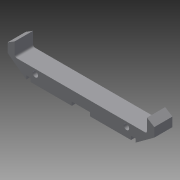
# Autodesk Inventor part: base
Saved by Autodesk Inventor 2014 SP1 (Build 180222100, 222)
## iProperties
Created: 2014-09-21
Part Number: base
Material: Générique
Document SubType Name: Modeling
Designer: astralien3000
Density: 1 g/cm^3
Appearance: Par défaut
Author: astralien3000
Autodesk Inventor part; units mm, degrees
ref_plane "YZ Plane" through (0, 0, 0) normal (1, 0, 0) x (0, 1, 0)
ref_plane "XZ Plane" through (0, 0, 0) normal (0, 1, 0) x (-1, 0, 0)
ref_plane "XY Plane" through (0, 0, 0) normal (0, 0, 1) x (1, 0, 0)
sketch "Esquisse1" plane through (0, 0, 0) normal (0, 1, 0) x (-1, 0, 0)
  circle A0 centre (0, 0) radius 25 construction
  line L0 (-25, 0) -> (25, 0) construction
  arc A1 (-75, -80.7775) -> (-75, 80.7775) centre (-25, 0) ccw construction
  arc A2 (75, 80.7775) -> (75, -80.7775) centre (25, 0) ccw construction
  line L1 (0, 25) -> (0, 0) construction
  line L2 (-75, 80.7775) -> (75, 80.7775)
  line L3 (-75, -80.7775) -> (75, -80.7775)
  arc A3 (75, -80.7775) -> (75, 80.7775) centre (25, 0) ccw
  arc A4 (-75, 80.7775) -> (-75, -80.7775) centre (-25, 0) ccw
  dimension "d0" = 50
  dimension "d1" = 190
  dimension "d2" = 150
  constraints: 11 point on circle, 8 end point, 5 centre point, 3 coincident, 2 perpendicular, 1 horizontal, 1 midpoint, 2 other
  measures "d0" diameter of A0
  measures "d1" diameter of A1
  measures "d2" distance of L2.start L2.end
extrude "Extrusion1" add sketch "Esquisse1" along normal mid plane 20
sketch "Esquisse4" plane through (0, -10, 0) normal (0, -1, 0) x (1, 0, 0)
  line L0 (-50, 40) -> (50, 40) construction
  line L1 (50, 40) -> (50, -40) construction
  line L2 (50, -40) -> (-50, -40) construction
  line L3 (-50, -40) -> (-50, 40) construction
  circle A0 centre (-50, 40) radius 3
  circle A1 centre (50, 40) radius 3
  circle A2 centre (50, -40) radius 3
  circle A3 centre (-50, -40) radius 3
  line L4 (75, 80.7775) -> (-75, 80.7775) projected
  point P0 (0, 0)
  dimension "d15" = 80
  dimension "d16" = 100
  dimension "d17" = 50
  dimension "d18" = 40
  dimension "d19" = 6
  dimension "d20" = 6
  dimension "d21" = 6
  dimension "d22" = 6
  dimension "d25" = 40.7775
  constraints: 8 end point, 4 centre point, 4 coincident, 2 parallel, 1 horizontal, 1 perpendicular
  measures "d15" distance of L0.end L1.end
  measures "d16" distance of L0.start L0.end
  measures "d17" distance from line of L1 point (0, 0)
  measures "d18" distance from line of L2 point (0, 0)
  measures "d19" diameter of A0
  measures "d20" diameter of A1
  measures "d21" diameter of A2
  measures "d22" diameter of A3
  measures "d25" distance between parallel lines of L4 L0
extrude "Extrusion4" cut sketch "Esquisse4" against normal through all
sketch "Esquisse12" plane through (0, -10, 0) normal (0, -1, 0) x (1, 0, 0)
  circle A0 centre (50, -40) radius 3 projected
  circle A1 centre (-50, 40) radius 3 projected
  circle A2 centre (50, 40) radius 3 projected
  circle A3 centre (-50, -40) radius 3 projected
  line L0 (75, 80.7775) -> (-75, 80.7775) projected
  arc A4 (-75, 80.7775) -> (-75, -80.7775) centre (-25, 0) ccw projected
  line L1 (-75, -80.7775) -> (75, -80.7775) projected
  arc A5 (75, -80.7775) -> (75, 80.7775) centre (25, 0) ccw projected
  line L2 (-72.5, 60) -> (72.5, 60)
  line L3 (72.5, 60) -> (72.5, 45)
  line L4 (72.5, 45) -> (-72.5, 45)
  line L5 (-72.5, 45) -> (-72.5, 60)
  line L6 (-60, 45) -> (60, 45)
  line L7 (60, 45) -> (60, 30)
  line L8 (60, 30) -> (-60, 30)
  line L9 (-60, 30) -> (-60, 45)
  line L10 (-72.5, 45) -> (-80.5, 45)
  line L11 (-80.5, 45) -> (-80.5, 55)
  line L12 (-80.5, 55) -> (-72.5, 55)
  line L13 (-72.5, 55) -> (-72.5, 45)
  line L14 (72.5, 45) -> (80.5, 45)
  line L15 (80.5, 45) -> (80.5, 55)
  line L16 (80.5, 55) -> (72.5, 55)
  line L17 (72.5, 55) -> (72.5, 45)
  line L18 (-60, 30) -> (-80.5, 45)
  line L19 (60, 30) -> (80.5, 45)
  line L20 (-80.5, 55) -> (-72.5, 60)
  line L21 (-72.5, 55) -> (-72.5, 60)
  line L22 (80.5, 55) -> (72.5, 60)
  line L23 (72.5, 60) -> (72.5, 55)
  line L24 (-60, 30) -> (-55, 30)
  line L25 (-55, 30) -> (-55, 34)
  line L26 (-55, 34) -> (-60, 34)
  line L27 (-60, 34) -> (-60, 30)
  line L28 (60, 30) -> (55, 30)
  line L29 (55, 30) -> (55, 34)
  line L30 (55, 34) -> (60, 34)
  line L31 (60, 34) -> (60, 30)
  line L32 (10, 30) -> (-10, 30)
  line L33 (-10, 30) -> (-10, 34)
  line L34 (-10, 34) -> (10, 34)
  line L35 (10, 34) -> (10, 30)
  point P0 (0, 0)
  dimension "d101" = 145
  dimension "d102" = 15
  dimension "d103" = 40.7775
  dimension "d105" = 72.5
  dimension "d106" = 10
  dimension "d107" = 10
  dimension "d108" = 10
  dimension "d109" = 8
  dimension "d110" = 8
  dimension "d111" = 5
  dimension "d112" = 5
  dimension "d116" = 5
  dimension "d117" = 4
  dimension "d118" = 5
  dimension "d119" = 4
  dimension "d120" = 4
  dimension "d121" = 20
  dimension "d122" = 10
  dimension "d144" = 5
  constraints: 68 end point, 15 parallel, 7 horizontal, 7 perpendicular, 2 point on line, 1 collinear
  measures "d101" distance of L2.start L2.end
  measures "d102" distance of L4.end L2.start
  measures "d103" distance from line of L0 A1.centre
  measures "d105" distance from line of point (0, 0) L5
  measures "d106" distance from line of L8 A1.centre
  measures "d107" distance from line of L9 A1.centre
  measures "d108" distance from line of L7 A2.centre
  measures "d109" distance between parallel lines of L13 L11
  measures "d110" distance between parallel lines of L3 L15
  measures "d111" distance between parallel lines of L2 L12
  measures "d112" distance between parallel lines of L2 L16
  measures "d116" distance between parallel lines of L27 L25
  measures "d117" distance between parallel lines of L8 L26
  measures "d118" distance from line of L7 L29.end
  measures "d119" distance between parallel lines of L8 L30
  measures "d120" distance between parallel lines of L32 L34
  measures "d121" distance between parallel lines of L35 L33
  measures "d122" distance from line of point (0, 0) L35
  measures "d144" distance from line of L6 A1.centre
extrude "Extrusion9" cut sketch "Esquisse12" against normal through all contours A5 L1 A4 L0 | L2 L3 L4 L5 | L9 L26 L25 L8 | L8 L29 L30 L7 | L33 L34 L35 L8
fillet "Congé1" radius 2 2 edges at (72.5, 0, 45) (-72.5, 0, 45)
equation "\"d17\" = 0.5 * d16"
equation "\"d18\" = 0.5 * d15"
equation "\"d20\" = d19"
equation "\"d21\" = d19"
equation "\"d22\" = d19"
